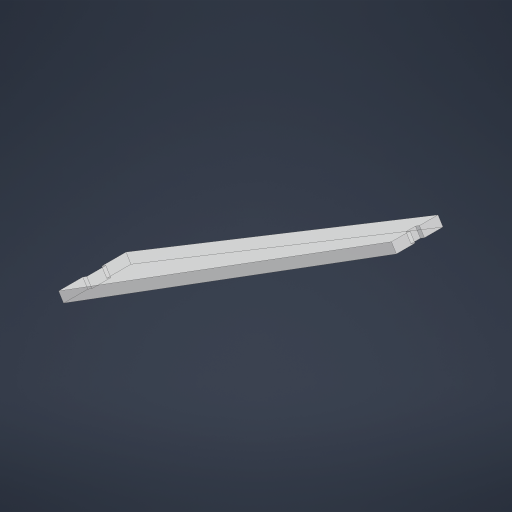
# Autodesk Inventor part: Touch Fifth
Saved by Autodesk Inventor 2023 (Build 270158000, 158)
## iProperties
Created: 2022-06-12
Part Number: Touch Fifth
Material: Polycarbonate, Smoke
Document SubType Name: Modeling
Designer: FizzyApple12
Density: 1.2 g/cm^3
Appearance: Polycarbonate - Semi Clear
Author: FizzyApple12
Autodesk Inventor part; units mm, degrees
ref_plane "XZ Plane" through (0, 0, 0) normal (0, 1, 0) x (-1, 0, 0)
ref_plane "XY Plane" through (0, 0, 0) normal (0, 0, 1) x (1, 0, 0)
sketch "Sketch1" plane through (0, 0, 0) normal (1, 0, 0) x (0, 1, 0)
  circle A0 centre (0, 0) radius 431.8 construction
  line L0 (-431.2082, -22.5987) -> (-431.2082, 22.5987)
  line L1 (-431.2082, -22.5987) -> (-386.0109, -22.5987) construction
  line L2 (-431.2082, -22.5987) -> (0, 0) construction
  line L3 (0, 0) -> (-431.2082, 22.5987) construction
  dimension "d0" = 863.6
  dimension "d3" = 90
  dimension "d4" = 6
  constraints: 8 end point, 2 point on circle, 1 centre point, 1 coincident, 1 horizontal, 1 perpendicular
  measures "d0" diameter of A0
  measures "d3" angle of L1 L0
  measures "d4" angle of L3 L2
ref_plane "Work Plane1" through (216.1794, 0, 0) normal (1, 0, 0) x (0, 1, 0)
sketch "Sketch2" plane through (216.1794, 0, 0) normal (1, 0, 0) x (0, 1, 0)
  circle A0 centre (0, 0) radius 298.45 construction
  line L0 (-298.041, 15.6197) -> (-298.041, -15.6197)
  line L1 (-298.041, 15.6197) -> (-266.8017, 15.6197) construction
  line L2 (-298.041, 15.6197) -> (0, 0) construction
  line L3 (0, 0) -> (-298.041, -15.6197) construction
  dimension "d2" = 596.9
  dimension "d5" = 90
  dimension "d6" = 6
  constraints: 8 end point, 2 point on circle, 1 centre point, 1 coincident, 1 horizontal, 1 perpendicular
  measures "d2" diameter of A0
  measures "d5" angle of L0 L1
  measures "d6" angle of L3 L2
ref_plane "Work Plane2" through (0, -431.2082, -22.5987) normal (-0.5244795, 0.8514231, 0) x (0, 0, 1)
sketch "Sketch3" plane through (0, -431.2082, -22.5987) normal (-0.5244795, 0.8514231, 0) x (0, 0, 1)
  line L0 (0, 0) -> (45.1973, 0) projected
  line L1 (38.2183, 253.9036) -> (6.979, 253.9036) projected
  line L2 (6.979, 253.9036) -> (0, 0)
  line L3 (45.1973, 0) -> (38.2183, 253.9036)
  point P0 (22.5987, 226.1599)
  constraints: 4 end point
extrude "Extrusion1" add sketch "Sketch3" against normal blind 6.35
sketch "Sketch5" plane through (0, -431.2082, -22.5987) normal (-0.5244795, 0.8514231, 0) x (0.8514231, 0.5244795, 0)
  line L0 (250.7286, -19.4237) -> (257.0786, -19.4237)
  line L1 (257.0786, -19.4237) -> (257.0786, -25.7737)
  line L2 (257.0786, -25.7737) -> (250.7286, -25.7737)
  line L3 (250.7286, -25.7737) -> (250.7286, -19.4237)
  line L4 (253.9036, -6.979) -> (253.9036, -38.2183) projected
  line L5 (250.7286, -19.4237) -> (257.0786, -25.7737) construction
  line L6 (257.0786, -19.4237) -> (250.7286, -25.7737) construction
  line L7 (-3.175, -28.9487) -> (3.175, -28.9487)
  line L8 (3.175, -28.9487) -> (3.175, -16.2487)
  line L9 (3.175, -16.2487) -> (-3.175, -16.2487)
  line L10 (-3.175, -16.2487) -> (-3.175, -28.9487)
  line L11 (0, -45.1973) -> (0, 0) projected
  line L12 (-3.175, -28.9487) -> (3.175, -16.2487) construction
  line L13 (3.175, -28.9487) -> (-3.175, -16.2487) construction
  point P0 (226.1599, -22.5987)
  point P1 (253.9036, -22.5987)
  point P2 (0, -22.5987)
  point P3 (0, -28.9487)
  point P4 (0, -16.2487)
  point P5 (253.9036, -19.4237)
  point P6 (253.9036, -25.7737)
  dimension "d15" = 6.35
  dimension "d16" = 6.35
  dimension "d17" = 6.35
  dimension "d18" = 12.7
  constraints: 24 end point, 6 midpoint, 4 parallel, 2 horizontal, 2 perpendicular
  measures "d15" distance of L1.end L2.end
  measures "d16" distance of L0.end L1.end
  measures "d17" distance of L9.end L8.end
  measures "d18" distance of L8.end L7.end
extrude "Extrusion3" cut sketch "Sketch5" against normal through all
body "Solid1"
